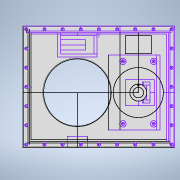
# Autodesk Inventor part: door top plate with window
Saved by Autodesk Inventor 2022 (Build 260153000, 153)
## iProperties
Created: 2021-11-30
Part Number: door top plate with window
Material: Generic
Document SubType Name: Modeling
Designer: a-dubs
Density: 1 g/cm^3
Appearance: Default
Author: a-dubs
Autodesk Inventor part; units mm, degrees
ref_plane "YZ Plane" through (0, 0, 0) normal (1, 0, 0) x (0, 1, 0)
ref_plane "XZ Plane" through (0, 0, 0) normal (0, 1, 0) x (-1, 0, 0)
ref_plane "XY Plane" through (0, 0, 0) normal (0, 0, 1) x (1, 0, 0)
sketch "Sketch1" plane through (0, 0, 0) normal (0, 1, 0) x (-1, 0, 0)
  line L0 (0, 0) -> (61, 0)
  circle A0 centre (0, 0) radius 33.6
  circle A1 centre (61, 0) radius 8.5
  line L1 (69.5, 0) -> (69.5, 7.5)
  line L2 (69.5, 7.5) -> (69.5, -7.5)
  line L3 (69.5, -7.5) -> (65, -7.5)
  line L4 (69.5, 7.5) -> (65, 7.5)
  line L5 (69.5, 7.5) -> (72.5, 7.5)
  line L6 (72.5, 7.5) -> (72.5, -7.5)
  line L7 (72.5, -7.5) -> (69.5, -7.5)
  line L8 (52.5, 0) -> (47.5, 0)
  line L9 (61, 8.5) -> (61, 13.5)
  line L10 (72.5, 0) -> (77.5, 0)
  line L11 (61, -8.5) -> (61, -13.5)
  line L12 (47.95, 13.05) -> (77.05, 13.05)
  line L13 (77.05, 13.05) -> (77.05, -13.05)
  line L14 (77.05, -13.05) -> (47.95, -13.05)
  line L15 (47.95, -13.05) -> (47.95, 13.05)
  line L16 (72.5, 7.5) -> (72.5, 10.5)
  line L17 (72.5, 10.5) -> (65, 10.5)
  line L18 (65, 10.5) -> (65, 7.5)
  line L19 (72.5, -7.5) -> (72.5, -10.5)
  line L20 (72.5, -10.5) -> (65, -10.5)
  line L21 (65, -10.5) -> (65, -7.5)
  line L22 (61, 0) -> (61, 60)
  line L23 (0, 0) -> (-42.65, 0)
  line L24 (-42.65, 0) -> (-47.65, 0)
  line L25 (0, 0) -> (0, -33.6)
  line L26 (0, 0) -> (42.65, 0)
  line L27 (42.65, 0) -> (42.65, 60)
  line L28 (42.65, 0) -> (42.65, -33.6)
  circle A2 centre (61, 0) radius 25
  line L29 (42.65, 25) -> (42.65, 31.2)
  line L30 (42.65, 31.2) -> (48.85, 31.2)
  line L31 (42.65, -25) -> (42.65, -31.2)
  line L32 (36, 0) -> (31, 0)
  line L33 (31, 0) -> (31, -31.2)
  line L34 (31, -31.2) -> (31, -37.4)
  line L35 (31, -37.4) -> (79.35, -37.4)
  line L36 (79.35, -37.4) -> (79.35, 31.2)
  line L37 (79.35, 31.2) -> (79.35, 37.4)
  line L38 (79.35, 37.4) -> (31, 37.4)
  line L39 (31, 37.4) -> (31, 0)
  line L40 (42.65, -33.6) -> (42.65, -37.4)
  circle A3 centre (61, 0) radius 5.25
  line L41 (86, 0) -> (91, 0)
  line L42 (91, 0) -> (97.4, 0)
  line L43 (-47.65, 0) -> (-47.65, 60)
  line L44 (-47.65, 60) -> (42.65, 60)
  line L45 (91, 0) -> (91, 60)
  line L46 (91, 60) -> (42.65, 60)
  line L47 (0, -33.6) -> (0, -43.6)
  line L48 (0, -43.6) -> (0, -48.6)
  line L49 (0, -48.6) -> (0, -55)
  line L50 (0, -55) -> (-54.05, -55)
  line L51 (0, -48.6) -> (-47.65, -48.6)
  line L52 (-47.65, -48.6) -> (-47.65, 0)
  line L53 (0, -55) -> (97.4, -55)
  line L54 (97.4, -55) -> (97.4, 0)
  line L55 (91, 0) -> (91, -48.6)
  line L56 (91, -48.6) -> (0, -48.6)
  line L57 (0, -48.6) -> (10, -48.6)
  line L58 (0, -48.6) -> (-10, -48.6)
  line L59 (10, -48.6) -> (10, -55)
  line L60 (-10, -48.6) -> (-10, -55)
  line L61 (10, -48.6) -> (10, -43.6)
  line L62 (10, -43.6) -> (-10, -43.6)
  line L63 (-10, -43.6) -> (-10, -49.0563)
  line L64 (65, 10.5) -> (66, 10.5)
  line L65 (66, 10.5) -> (66, 7.5)
  line L66 (65, -10.5) -> (66, -10.5)
  line L67 (66, -10.5) -> (66, -7.5)
  line L68 (-47.65, 0) -> (-54.05, 0)
  line L69 (42.65, 60) -> (42.65, 66.4)
  line L70 (-54.05, -55) -> (-54.05, 0)
  line L71 (-54.05, 66.4) -> (-54.05, 0)
  line L72 (42.65, 66.4) -> (-54.05, 66.4)
  line L73 (97.4, 0) -> (97.4, 66.4)
  line L74 (97.4, 66.4) -> (42.65, 66.4)
  line L75 (-47.65, 60) -> (-50.85, 60)
  line L76 (-50.85, 60) -> (-50.85, 63.2)
  circle A4 centre (-50.85, 63.2) radius 1.6
  line L77 (91, 60) -> (94.2, 60)
  line L78 (94.2, 60) -> (-50.85, 60)
  circle A5 centre (-32.7188, 63.2) radius 1.6
  circle A6 centre (-14.5875, 63.2) radius 1.6
  circle A7 centre (3.5438, 63.2) radius 1.6
  circle A8 centre (21.675, 63.2) radius 1.6
  circle A9 centre (39.8063, 63.2) radius 1.6
  circle A10 centre (57.9375, 63.2) radius 1.6
  circle A11 centre (76.0688, 63.2) radius 1.6
  circle A12 centre (94.2, 63.2) radius 1.6
  line L79 (-47.65, 60) -> (-47.65, 63.2)
  line L80 (-47.65, 63.2) -> (-47.65, -51.8)
  circle A13 centre (-50.85, 44.0333) radius 1.6
  circle A14 centre (-50.85, 24.8667) radius 1.6
  circle A15 centre (-50.85, 5.7) radius 1.6
  circle A16 centre (-50.85, -13.4667) radius 1.6
  circle A17 centre (-50.85, -32.6333) radius 1.6
  circle A18 centre (-50.85, -51.8) radius 1.6
  line L81 (-47.65, 60) -> (21.675, 60)
  line L82 (21.675, 60) -> (21.675, 55.1722)
  line L83 (-47.65, 5.7) -> (-45.15, 5.7)
  circle A19 centre (-50.85, -51.8) radius 1.6
  circle A20 centre (-32.7188, -51.8) radius 1.6
  circle A21 centre (-14.5875, -51.8) radius 1.6
  circle A22 centre (3.5438, -51.8) radius 1.6
  circle A23 centre (21.675, -51.8) radius 1.6
  circle A24 centre (39.8063, -51.8) radius 1.6
  circle A25 centre (57.9375, -51.8) radius 1.6
  circle A26 centre (76.0688, -51.8) radius 1.6
  circle A27 centre (94.2, -51.8) radius 1.6
  circle A28 centre (94.2, 44.0333) radius 1.6
  circle A29 centre (94.2, 24.8667) radius 1.6
  circle A30 centre (94.2, 5.7) radius 1.6
  circle A31 centre (94.2, -13.4667) radius 1.6
  circle A32 centre (94.2, -32.6333) radius 1.6
  line L84 (61, 60) -> (61, 56.8)
  line L85 (61, 56.8) -> (61, 38.8)
  line L86 (61, 56.8) -> (48.1, 56.8)
  line L87 (61, 56.8) -> (73.9, 56.8)
  line L88 (73.9, 56.8) -> (73.9, 38.8)
  line L89 (73.9, 38.8) -> (61, 38.8)
  line L90 (48.1, 56.8) -> (48.1, 38.8)
  line L91 (48.1, 38.8) -> (61, 38.8)
  line L92 (0, 60) -> (0, 56.8)
  line L93 (0, 56.8) -> (-16.65, 56.8)
  line L94 (-16.65, 56.8) -> (16.65, 56.8)
  line L95 (16.65, 56.8) -> (16.65, 38.6)
  line L96 (16.65, 38.6) -> (-16.65, 38.6)
  line L97 (-16.65, 38.6) -> (-16.65, 56.8)
  circle A33 centre (-50.85, 63.2) radius 1.4
  circle A34 centre (-32.7188, 63.2) radius 1.4
  circle A35 centre (-14.5875, 63.2) radius 1.4
  circle A36 centre (3.5438, 63.2) radius 1.4
  circle A37 centre (21.675, 63.2) radius 1.4
  circle A38 centre (39.8063, 63.2) radius 1.4
  circle A39 centre (57.9375, 63.2) radius 1.4
  circle A40 centre (76.0688, 63.2) radius 1.4
  circle A41 centre (94.2, 63.2) radius 1.4
  circle A42 centre (-50.85, -51.8) radius 1.4
  circle A43 centre (-32.7188, -51.8) radius 1.4
  circle A44 centre (-14.5875, -51.8) radius 1.4
  circle A45 centre (3.5438, -51.8) radius 1.4
  circle A46 centre (21.675, -51.8) radius 1.4
  circle A47 centre (39.8063, -51.8) radius 1.4
  circle A48 centre (57.9375, -51.8) radius 1.4
  circle A49 centre (76.0688, -51.8) radius 1.4
  circle A50 centre (94.2, -51.8) radius 1.4
  circle A51 centre (-50.85, 44.0333) radius 1.4
  circle A52 centre (-50.85, 24.8667) radius 1.4
  circle A53 centre (-50.85, 5.7) radius 1.4
  circle A54 centre (-50.85, -13.4667) radius 1.4
  circle A55 centre (-50.85, -32.6333) radius 1.4
  circle A56 centre (-50.85, -51.8) radius 1.4
  circle A57 centre (94.2, 63.2) radius 1.4
  circle A58 centre (94.2, 44.0333) radius 1.4
  circle A59 centre (94.2, 24.8667) radius 1.4
  circle A60 centre (94.2, 5.7) radius 1.4
  circle A61 centre (94.2, -13.4667) radius 1.4
  circle A62 centre (94.2, -32.6333) radius 1.4
  circle A63 centre (94.2, -51.8) radius 1.4
  line L98 (61, 8.5) -> (61, 6.7)
  line L99 (61, 6.7) -> (61.8, 6.7)
  line L100 (61, 6.7) -> (60.2, 6.7)
  line L101 (60.2, 6.7) -> (60.2, 8.4623)
  line L102 (61.8, 6.7) -> (61.8, 8.4623)
  line L103 (-16.65, 56.8) -> (-16.65, 60)
  line L104 (-16.65, 60) -> (-19.85, 60)
  line L105 (16.65, 38.6) -> (19.85, 38.6)
  line L106 (19.85, 38.6) -> (19.85, 35.4)
  line L107 (-19.85, 60) -> (19.85, 60)
  line L108 (19.85, 60) -> (19.85, 35.4)
  line L109 (19.85, 35.4) -> (-19.85, 35.4)
  line L110 (-19.85, 35.4) -> (-19.85, 60)
  line L111 (-16.65, 47.7) -> (8.35, 47.7)
  line L112 (16.65, 56.8) -> (19.85, 56.8)
  line L113 (16.65, 38.6) -> (19.85, 38.6)
  line L114 (8.35, 47.7) -> (8.35, 52.7)
  line L115 (8.35, 47.7) -> (8.35, 42.7)
  line L116 (8.35, 42.7) -> (-16.65, 42.7)
  line L117 (8.35, 52.7) -> (-16.65, 52.7)
  line L118 (79.35, -37.4) -> (82.55, -37.4)
  line L119 (82.55, -37.4) -> (82.55, 37.4)
  line L120 (82.55, 37.4) -> (79.35, 37.4)
  line L121 (48.85, 31.2) -> (45.65, 31.2)
  circle A64 centre (45.65, 31.2) radius 1.6
  circle A65 centre (45.65, 31.2) radius 1.4
  circle A66 centre (45.65, 31.2) radius 3.2
  circle A67 centre (76.35, 31.2) radius 1.6
  circle A68 centre (76.35, 31.2) radius 1.4
  circle A69 centre (76.35, 31.2) radius 3.2
  circle A70 centre (45.65, -31.2) radius 1.6
  circle A71 centre (45.65, -31.2) radius 1.4
  circle A72 centre (45.65, -31.2) radius 3.2
  circle A73 centre (76.35, -31.2) radius 3.2
  circle A74 centre (76.35, -31.2) radius 1.6
  circle A75 centre (76.35, -31.2) radius 1.4
  line L122 (91, -48.6) -> (92.6, -48.6)
  line L123 (92.6, -48.6) -> (92.6, -50.2)
  line L124 (-47.65, 60) -> (-49.25, 60)
  line L125 (-49.25, 60) -> (-49.25, 61.6)
  line L126 (-47.65, 60) -> (-46.05, 60)
  line L127 (-46.05, 60) -> (-46.05, 58.4)
  line L128 (91, -48.6) -> (89.4, -48.6)
  line L129 (89.4, -48.6) -> (89.4, -47)
  line L130 (89.4, -47) -> (-46.05, -47)
  line L131 (-46.05, -47) -> (-46.05, 58.4)
  line L132 (-46.05, 58.4) -> (89.4, 58.4)
  line L133 (89.4, 58.4) -> (89.4, -47)
  line L134 (-49.25, 61.6) -> (92.6, 61.6)
  line L135 (92.6, 61.6) -> (92.6, -50.2)
  line L136 (92.6, -50.2) -> (-49.25, -50.2)
  line L137 (-49.25, -50.2) -> (-49.25, 61.6)
  point P0 (42.65, 37.4)
  point P1 (31, -12.9599)
  point P2 (31, 12.9599)
  dimension "d1" = 67.2
  dimension "d2" = 17
  dimension "d0" = 61
  dimension "d3" = 7.5
  dimension "d4" = 15
  dimension "d5" = 3
  dimension "d6" = 5
  dimension "d7" = 5
  dimension "d8" = 5
  dimension "d9" = 5
  dimension "d10" = 3
  dimension "d11" = 60
  dimension "d13" = 42.65
  dimension "d14" = 5
  dimension "d16" = 50
  dimension "d17" = 6.2
  dimension "d18" = 6.2
  dimension "d19" = 6.2
  dimension "d26" = 5
  dimension "d27" = 6.2
  dimension "d31" = 10.5
  dimension "d33" = 5
  dimension "d34" = 6.4
  dimension "d36" = 10
  dimension "d37" = 5
  dimension "d38" = 6.4
  dimension "d41" = 10
  dimension "d42" = 10
  dimension "d52" = 1
  dimension "d53" = 1
  dimension "d56" = 6.4
  dimension "d57" = 6.4
  dimension "d58" = 3.2
  dimension "d59" = 3.2
  dimension "d62" = 18.1313
  dimension "d67" = 115
  dimension "d70" = 19.1667
  dimension "d78" = 3.2
  dimension "d79" = 18
  dimension "d80" = 12.9
  dimension "d81" = 12.9
  dimension "d82" = 3.2
  dimension "d83" = 16.65
  dimension "d84" = 33.3
  dimension "d85" = 18.2
  dimension "d93" = 2.8
  dimension "d96" = 18.1313
  dimension "d99" = 115
  dimension "d104" = 19.1667
  dimension "d107" = 145.05
  dimension "d110" = 1.8
  dimension "d111" = 0.8
  dimension "d112" = 0.8
  dimension "d115" = 3.2
  dimension "d116" = 3.2
  dimension "d117" = 3.2
  dimension "d118" = 3.2
  dimension "d119" = 25
  dimension "d120" = 5
  dimension "d121" = 5
  dimension "d127" = 3.2
  dimension "d128" = 3.2
  dimension "d129" = 2.8
  dimension "d130" = 6.4
  dimension "d137" = 1.6
  dimension "d138" = 1.6
  constraints: 276 end point, 74 centre point, 44 point on line, 43 perpendicular, 26 symmetric about line, 24 horizontal, 23 vertical, 16 coincident, 14 parallel, 4 collinear, 4 midpoint, 2 point on circle, 124 other
  measures "d0" distance of L0.start L0.end
  measures "d3" distance of L1.start L1.end
  measures "d4" distance of L1.end L2.end
  measures "d5" distance of L1.end L5.end
  measures "d6" distance of L8.start L8.end
  measures "d7" distance of L9.start L9.end
  measures "d8" distance of L10.start L10.end
  measures "d9" distance of L11.start L11.end
  measures "d10" distance of L5.end L16.end
  measures "d11" distance of L22.start L22.end
  measures "d13" distance of L23.start L23.end
  measures "d14" distance of L23.end L24.end
  measures "d16" diameter of A2
  measures "d17" distance of L29.start L29.end
  measures "d18" distance of L29.end L30.end
  measures "d19" distance of L31.start L31.end
  measures "d26" distance of L32.start L32.end
  measures "d27" distance of L33.end L34.end
  measures "d31" diameter of A3
  measures "d33" distance of L41.start L41.end
  measures "d34" distance of L41.end L42.end
  measures "d36" distance of L25.end L47.end
  measures "d37" distance of L47.end L48.end
  measures "d38" distance of L48.end L49.end
  measures "d41" distance of L48.end L57.end
  measures "d42" distance of L48.end L58.end
  measures "d52" distance of L17.end L64.end
  measures "d53" distance of L20.end L66.end
  measures "d56" distance of L24.end L68.end
  measures "d57" distance of L27.end L69.end
  measures "d58" distance of L43.end L75.end
  measures "d59" diameter of A4
  measures "d62" distance of A4.centre A5.centre
  measures "d67" distance of L79.end L80.end
  measures "d70" distance of A4.centre A13.centre
  measures "d78" distance of L22.end L84.end
  measures "d79" distance of L84.end L85.end
  measures "d80" distance of L84.end L86.end
  measures "d81" distance of L84.end L87.end
  measures "d82" distance of L92.start L92.end
  measures "d83" distance of L92.end L93.end
  measures "d84" distance of L93.end L94.end
  measures "d85" distance of L94.end L95.end
  measures "d93" diameter of A33
  measures "d96" distance of A33.centre A34.centre
  measures "d99" distance of A33.centre A42.centre
  measures "d104" distance of A33.centre A51.centre
  measures "d107" distance of A33.centre A57.centre
  measures "d110" distance of L9.start L98.end
  measures "d111" distance of L98.end L99.end
  measures "d112" distance of L98.end L100.end
  measures "d115" distance of L93.end L103.end
  measures "d116" distance of L103.end L104.end
  measures "d117" distance of L95.end L105.end
  measures "d118" distance of L105.end L106.end
  measures "d119" distance of L111.start L111.end
  measures "d120" distance of L111.end L114.end
  measures "d121" distance of L111.end L115.end
  measures "d127" distance of L121.start L121.end
  measures "d128" diameter of A64
  measures "d129" diameter of A65
  measures "d130" diameter of A66
  measures "d137" distance of L122.end L123.end
  measures "d138" distance of L43.end L124.end
extrude "backplate" add sketch "Sketch1" against normal blind 3.2 contours L23 L24 L131 L132 L110 L109 L106 L108 L27 L38 L39 A0 | A0 L47 L62 L63 L130 L131 L24 L23 | A0 L33 L34 L35 L118 L119 A2 L41 L133 L130 L61 L62 L47 | A0 L39 L38 L27 A66 A2 L0 | L0 A2 L28 A72 L40 L35 L34 L33 A0 | L62 L61 L130 L48 | L48 L130 L63 L62 | A2 L27 L0 | L0 L28 A2 | L131 L130 L63 L51 L52 L24 | L24 L43 L83 L131 | L130 L61 L56 L48 | L48 L51 L63 L130 | L27 A2 L22 L9 L12 L15 L0 | L0 L15 L14 L13 L12 L9 L22 A2 L36 L28 | L27 A66 L38 L22 A2 | A2 L36 A73 L35 L40 L28 A72 | L27 L132 L22 L86 L90 L91 L38 | L68 L137 L75 L43 | L52 L80 L136 L137 L68 | L83 L43 L44 L127 L131 | L56 L59 L136 L49 | L49 L136 L60 L51 | L130 L129 L56 L61 | L22 L38 L37 A69 L36 A2 | L36 A2 L119 | A2 L119 L118 L36 A73 | A66 L30 A64 L27 | L27 A66 | L132 L82 L44 L27 | L27 L46 L22 L132 | L22 L89 L88 L87 L132 L133 L41 A2 L119 L120 L38 | L51 L60 L136 L80 | A21 | A20 | A17 | A16 | L137 L136 L60 L50 L70 L68 | A15 | A14 | A13 | A5 | A6 | A7 | A8 | A9 | L68 L71 L72 L69 L134 L125 L137 | L127 L44 L110 L132 | A22 | L136 L59 L53 L49 | L49 L50 L60 L136 | L56 L122 L123 L136 L59 | L133 L41 L55 L56 L129 | L15 L12 L9 A1 L0 | L0 A1 L11 L14 L15 | L27 L30 A64 A66 | L36 A69 L37 L120 L119 A2 | A72 L28 | L28 A72 | L119 A2 | A73 L36 | L36 A73 | L69 L134 L135 L77 L46 | L44 L79 L134 L69 | L132 L108 L44 L82 | L22 L46 L45 L41 L133 L132 | L91 L90 L86 L22 | L22 L87 L88 L89 | L75 L125 L134 L79 | L132 L103 L97 L96 L105 L106 L109 L110 | L110 L44 L103 L132 | A31 | A32 | A26 | A25 | A24 | A23 | L136 L123 L135 L42 L54 L53 L59 | A1 L101 L100 L22 A3 L0 | L0 A3 L22 L99 L102 A1 | L12 L13 L10 L6 L16 L17 L18 A1 L9 | A69 L37 L36 | L36 L37 A69 | A64 L30 A65 | L30 A65 A64 | A10 | A11 | A28 | A29 | A30 | L69 L74 L73 L42 L135 L134 | L132 L92 L44 L108 | L108 L112 L94 L92 L132 | L132 L92 L93 L103 | L103 L44 L92 L132 | L55 L42 L135 L122 | L45 L77 L135 L42 | A3 L22 L0 | L0 L22 A3 | A1 L22 L100 L101 | A1 L21 L20 L19 L6 L10 L13 L14 L11 | A1 L102 L99 L22 | A65 L30 | L30 A65 | L108 L105 L95 L112 | L93 L94 L95 L96 L97 L116 L115 L114 L117 | A1 L2 L3 | L3 L67 L20 L21 | L117 L114 L111 L97 | A1 L4 L1 | L1 L5 L6 L7 L2 | L3 L7 L19 L20 L67 | L18 L17 L65 L4 | L111 L115 L116 L97 | L4 L65 L17 L16 L5 | A4 | A12 | A18 | A27 | A33 | A34 | A35 | A36 | A37 | A38 | A39 | A40 | A41 | A42 | A43 | A44 | A45 | A46 | A47 | A48 | A49 | A50 | A51 | A52 | A53 | A54 | A55 | A58 | A59 | A60 | A61 | A62 | A67 | A68 | A70 | A71 | A74 | A75
fillet "Fillet3" radius 3.2 4 edges at (54.05, -1.6, -55) (-97.4, -1.6, -55) (-97.4, -1.6, 66.4) (54.05, -1.6, 66.4)
extrude "B2 male pegs" cut sketch "Sketch1" against normal through all contours A4 | A12 | A18 | A27 | A33 | A41 | A42 | A50
fillet "Fillet8" radius 0.8 8 edges at (-96.4627, 0, -54.0627) (-97.4, 0, 5.7) (-96.4627, 0, 65.4627) (-21.675, 0, 66.4) (53.1127, 0, 65.4627) (54.05, 0, 5.7) (53.1127, 0, -54.0627) (-21.675, 0, -55)
extrude "Extrusion12" cut sketch "Sketch1" along normal blind 2.4 from surface at -3.2 contours L23 A0 L39 L0 | L25 A0 L23 | L0 L33 A0 L25 | L39 A0 L0 | L0 A0 L33 | L23 L24 L131 L132 L110 L109 L106 L108 L27 L38 L39 A0 | A0 L47 L62 L63 L130 L131 L24 L23 | A0 L33 L34 L35 L118 L119 A2 L41 L133 L130 L61 L62 L47 | A0 L39 L38 L27 A66 A2 L0 | L0 A2 L28 A72 L40 L35 L34 L33 A0 | L62 L61 L130 L48 | L48 L130 L63 L62 | A2 L27 L0 | L0 L28 A2 | L131 L130 L63 L51 L52 L24 | L24 L43 L83 L131 | L130 L61 L56 L48 | L48 L51 L63 L130 | L27 A2 L22 L9 L12 L15 L0 | L0 L15 L14 L13 L12 L9 L22 A2 L36 L28 | L27 A66 L38 L22 A2 | A2 L36 A73 L35 L40 L28 A72 | L27 L132 L22 L86 L90 L91 L38 | L68 L137 L75 L43 | L52 L80 L136 L137 L68 | L83 L43 L44 L127 L131 | L56 L59 L136 L49 | L49 L136 L60 L51 | L130 L129 L56 L61 | L22 L38 L37 A69 L36 A2 | L36 A2 L119 | A2 L119 L118 L36 A73 | A66 L30 A64 L27 | L27 A66 | L132 L82 L44 L27 | L27 L46 L22 L132 | L22 L89 L88 L87 L132 L133 L41 A2 L119 L120 L38 | L51 L60 L136 L80 | L127 L44 L110 L132 | L56 L122 L123 L136 L59 | L133 L41 L55 L56 L129 | L15 L12 L9 A1 L0 | L0 A1 L11 L14 L15 | L27 L30 A64 A66 | L36 A69 L37 L120 L119 A2 | A72 L28 | L28 A72 | L119 A2 | A73 L36 | L36 A73 | L69 L134 L135 L77 L46 | L44 L79 L134 L69 | L132 L108 L44 L82 | L22 L46 L45 L41 L133 L132 | L91 L90 L86 L22 | L22 L87 L88 L89 | L75 L125 L134 L79 | L132 L103 L97 L96 L105 L106 L109 L110 | L110 L44 L103 L132 | A1 L101 L100 L22 A3 L0 | L0 A3 L22 L99 L102 A1 | L12 L13 L10 L6 L16 L17 L18 A1 L9 | A69 L37 L36 | L36 L37 A69 | A64 L30 A65 | L30 A65 A64 | L132 L92 L44 L108 | L108 L112 L94 L92 L132 | L132 L92 L93 L103 | L103 L44 L92 L132 | L55 L42 L135 L122 | L45 L77 L135 L42 | A3 L22 L0 | L0 L22 A3 | A1 L22 L100 L101 | A1 L21 L20 L19 L6 L10 L13 L14 L11 | A1 L102 L99 L22 | A65 L30 | L30 A65 | L108 L105 L95 L112 | L93 L94 L95 L96 L97 L116 L115 L114 L117 | A1 L2 L3 | L3 L67 L20 L21 | L117 L114 L111 L97 | A1 L4 L1 | L1 L5 L6 L7 L2 | L3 L7 L19 L20 L67 | L18 L17 L65 L4 | L111 L115 L116 L97 | L4 L65 L17 L16 L5 | A67 | A68 | A70 | A71 | A74 | A75
fillet "Fillet10" radius 0.8 1 edges at (33.6, 0, 0)
body "Solid2"
